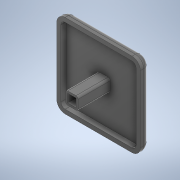
# Autodesk Inventor part: Abdeckkappe 5 20x20
Saved by Autodesk Inventor 2021 (Build 250183000, 183)
## iProperties
Created: 2021-05-07
Part Number: Abdeckkappe 5 20x20
Material: Generisch
Document SubType Name: Modeling
Designer: Sebastian Seewald
Mass: 0.490912 g
Surface Area: 11.617 cm^2
Volume: 0.490912 cm^3
Density: 1 g/cm^3
Appearance: Vorgabe
Author: Sebastian Seewald
Autodesk Inventor part; units mm, degrees
ref_plane "YZ Plane" through (0, 0, 0) normal (1, 0, 0) x (0, 1, 0)
ref_plane "XZ Plane" through (0, 0, 0) normal (0, 1, 0) x (-1, 0, 0)
ref_plane "XY Plane" through (0, 0, 0) normal (0, 0, 1) x (1, 0, 0)
sketch "Skizze1" plane through (0, 0, 0) normal (0, 0, 1) x (1, 0, 0)
  line L0 (-10, 10) -> (10, 10)
  line L1 (10, 10) -> (10, -10)
  line L2 (10, -10) -> (-10, -10)
  line L3 (-10, -10) -> (-10, 10)
  line L4 (-10, 10) -> (10, -10) construction
  line L5 (10, 10) -> (-10, -10) construction
  point P0 (0, 0)
  dimension "d0" = 20
  dimension "d1" = 20
  constraints: 12 end point, 2 midpoint, 2 parallel, 1 horizontal, 1 perpendicular
  measures "d0" distance of L0.start L0.end
  measures "d1" distance of L2.end L0.start
extrude "Extrusion1" add sketch "Skizze1" along normal blind 2.3
fillet "Rundung1" radius 2 4 edges at (10, 10, 1.15) (-10, 10, 1.15) (10, -10, 1.15) (-10, -10, 1.15)
shell "Wandung1" thickness 1 removed faces 1 at (-2.6667, -2, 2.3)
fillet "Rundung2" radius 1.5 8 edges at (-9.4142, 9.4142, 0) (-10, 0, 0) (-9.4142, -9.4142, 0) (0, -10, 0) (9.4142, -9.4142, 0) (10, 0, 0) (9.4142, 9.4142, 0) (0, 10, 0)
sketch "Skizze2" plane through (-9, 9, 1) normal (0, 0, 1) x (1, 0, 0)
  line L0 (7.5, -7.5) -> (10.5, -7.5)
  line L1 (10.5, -7.5) -> (10.5, -10.5)
  line L2 (10.5, -10.5) -> (7.5, -10.5)
  line L3 (7.5, -10.5) -> (7.5, -7.5)
  line L4 (7.5, -7.5) -> (10.5, -10.5) construction
  line L5 (10.5, -7.5) -> (7.5, -10.5) construction
  point P0 (9, -9)
  dimension "d7" = 3
  dimension "d8" = 3
  constraints: 12 end point, 2 midpoint, 2 parallel, 1 horizontal, 1 perpendicular
  measures "d7" distance of L0.start L0.end
  measures "d8" distance of L2.end L0.start
extrude "Extrusion2" add sketch "Skizze2" along normal blind 7.7
fillet "Rundung3" radius 0.5 4 edges at (1.5, 1.5, 4.85) (-1.5, 1.5, 4.85) (1.5, -1.5, 4.85) (-1.5, -1.5, 4.85)
shell "Wandung2" thickness 0.5 removed faces 1 at (0.3333, -0.5, 8.7)
